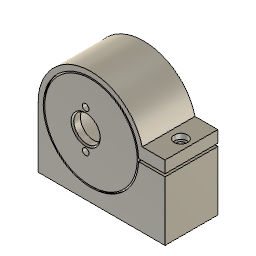
ワインダー量産試作機外装作成前配置 (Autodesk Fusion 360 archive; units mm, degrees)
design "モーターマウント"
Autodesk Fusion 360 part; units mm, degrees
note: some values were not read from the file. Chosen so that the rebuilt part matches the saved one: that a step has no effect. Set by a fixed rule: which sketch regions a step uses.
sketch "スケッチ1" plane through (0, 0, 0) normal (0, 1, 0) x (1, 0, 0)
  line L0 (0, 20) -> (0, 18)
  line L1 (20, -5) -> (28, -5)
  line L2 (20, -5) -> (19.3649, -5)
  line L3 (-20, 23) -> (0, 23)
  line L4 (0, 20) -> (0, 18)
  line L5 (28, 18) -> (28, 23)
  line L6 (28, 23) -> (0, 23)
  line L7 (0, 20) -> (0, 18)
  line L8 (-20, 0) -> (-20, 18)
  arc A0 (-20, 0) -> (19.3649, -5) centre (0, 0) ccw
  line L9 (-20, 18) -> (-20, 23)
  line L10 (28, -0.5) -> (17.9931, -0.5)
  line L11 (17.9931, 0.5) -> (28, 0.5)
  arc A1 (17.9931, 0.5) -> (17.9931, -0.5) centre (0, 0) ccw
  line L12 (28, -5) -> (28, -0.5)
  line L13 (28, 0.5) -> (28, 20)
  dimension "d1" = 36
  dimension "d4" = 5
  constraint coincident A0.centre A1.centre
  constraint vertical L0
  constraint perpendicular L1 L12
  constraint horizontal L3
  constraint vertical L4
  constraint coincident L0.end A1
  constraint vertical L5
  constraint horizontal L6
  constraint vertical L7
  constraint perpendicular L3 L9
  constraint coincident L11.end L12
  constraint perpendicular L11 L12
  constraint collinear L12 L13
  measures "d1" diameter of A1
  measures "d4" distance of L0.end L3.end
extrude "押し出し1" add sketch "スケッチ1" along normal blind 20 makes body 1
sketch "スケッチ2" plane through (0, 0, 5) normal (0, 0, 1) x (-1, 0, 0)
  line L0 (-19.3649, 0) -> (-28, 0)
  line L1 (-28, 0) -> (-28, -20)
  line L2 (-28, -20) -> (-19.3649, -20)
  line L3 (-19.3649, -20) -> (-19.3649, 0)
  circle A0 centre (-24, -10) radius 2.5
  dimension "d7" = 5
  measures "d7" diameter of A0
extrude "押し出し2" cut sketch "スケッチ2" against normal blind 2 contours A0 bodies 1
sketch "スケッチ3" plane through (0, 0, 3) normal (0, 0, 1) x (-1, 0, 0)
  circle A0 centre (-24, -10) radius 2.5
  circle A1 centre (-24, -10) radius 1.5
  dimension "d10" = 3
  constraint concentric A0 A1
  measures "d10" diameter of A1
extrude "押し出し3" cut sketch "スケッチ3" against normal blind 26 contours A1 bodies 1
sketch "スケッチ5" plane through (0, 0, 0) normal (0, 1, 0) x (1, 0, 0)
  line L0 (28, 23) -> (-20, 23)
  line L1 (-20, 23) -> (-20, 19)
  line L2 (-20, 19) -> (28, 19)
  line L3 (28, 19) -> (28, 23)
  constraint horizontal L0
  constraint vertical L1
  constraint horizontal L2
  constraint vertical L3
sketch "スケッチ8" plane through (0, 0, -23) normal (0, 0, -1) x (1, 0, 0)
  line L0 (0, -20) -> (0, 0)
  line L1 (-20, 0) -> (-20, -20)
  line L2 (28, -10) -> (24, -10)
  line L3 (26.8, -8.3834) -> (24, -6.7668)
  line L4 (24, -6.7668) -> (21.2, -8.3834)
  line L5 (21.2, -8.3834) -> (21.2, -11.6166)
  line L6 (21.2, -11.6166) -> (24, -13.2332)
  line L7 (24, -13.2332) -> (26.8, -11.6166)
  line L8 (26.8, -11.6166) -> (26.8, -8.3834)
  line L9 (0, 0) -> (-20, 0)
  line L10 (-20, -20) -> (0, -20)
  point P0 (24, -10)
  dimension "d20" = 4
  dimension "d21" = 2.8
  constraint coincident P0 L2.end
  measures "d20" distance of L2.start P0
  measures "d21" distance of P0 L8
extrude "押し出し6" cut sketch "スケッチ8" against normal blind 15 contours L3 L4 L5 L6 L7 L8 bodies 1
extrude "押し出し7" [no effect]
sketch "スケッチ15" plane through (0, 0, -23) normal (0, 0, -1) x (1, 0, 0)
  line L0 (24, -6.7668) -> (26.8, -8.3834)
  line L1 (26.8, -8.3834) -> (26.8, -11.6166)
  line L2 (26.8, -11.6166) -> (24, -13.2332)
  line L3 (24, -13.2332) -> (21.2, -11.6166)
  line L4 (21.2, -11.6166) -> (21.2, -8.3834)
  line L5 (21.2, -8.3834) -> (24, -6.7668)
  line L6 (28, 0) -> (0, 0)
  line L7 (0, 0) -> (0, -20)
  line L8 (0, -20) -> (28, -20)
  line L9 (28, -20) -> (28, 0)
  point P0 (25, -17)
  point P1 (-17, -17)
  point P2 (-17, -3)
  point P3 (25, -3)
hole "穴2" at (25, 17, -23) at (25, 3, -23) at (-17, 3, -23) at (-17, 17, -23) direction (0, 0, 1) diameter 2.5 depth 5 tip angle 180 bodies 1
sketch "スケッチ1 (2)" plane through (0, 0, 0) normal (0, 1, 0) x (1, 0, 0) in component "モーターマウント(内部) v1"
  circle A0 centre (0, 0) radius 18
  circle A1 centre (-2, 0) radius 13.85
  dimension "d5_1" = 27.7
  constraint coincident A0.centre origin
  measures "d5_1" diameter of A1
extrude "押し出し2'" add sketch "スケッチ1 (2)" along normal blind 20 separate body makes body 2 in component "モーターマウント(内部) v1"
sketch "スケッチ2 (2)" plane through (0, 0, 0) normal (0, 1, 0) x (1, 0, 0) in component "モーターマウント(内部) v1"
  circle A0 centre (-2, 0) radius 13.85
  circle A1 centre (-2, 0) radius 5
  dimension "d8_1" = 27.7
  dimension "d11_1" = 10
  constraint concentric A0 A1
  measures "d8_1" diameter of A0
  measures "d11_1" diameter of A1
extrude "押し出し4" add sketch "スケッチ2 (2)" along normal blind 3 bodies 2 in component "モーターマウント(内部) v1"
sketch "スケッチ3 (2)" plane through (0, 0, 0) normal (0, -1, 0) x (1, 0, 0) in component "モーターマウント(内部) v1"
  circle A0 centre (-2, 0) radius 5
  circle A1 centre (0, 0) radius 18
  circle A2 centre (-2, -7.25) radius 1.25
  line L0 (-2, 0) -> (-2, 7.25)
  circle A3 centre (-2, 7.25) radius 1.25
  point P0 (-2, 0)
  dimension "d14" = 7.25
  dimension "d15" = 2.5
  dimension "d16" = 7.25
  dimension "d17" = 2.5
  constraint coincident P0 A0.centre
  constraint vertical L0
  constraint coincident L0.end A3.centre
  measures "d14" distance of P0 A2.centre
  measures "d15" diameter of A2
  measures "d16" distance of P0 L0.end
  measures "d17" diameter of A3
extrude "押し出し5" cut sketch "スケッチ3 (2)" against normal blind 3 contours A2 | A3 bodies 2 in component "モーターマウント(内部) v1"
chamfer "面取り1" distance 0.5 angle 45 2 edges at (-16.7819, 0, 6.5091) (-6.6616, 0, -1.8081) on bodies 2 in component "モーターマウント(内部) v1"
chamfer "面取り2" distance 0.5 angle 45 2 edges at (-16.7819, 20, 6.5091) (-14.9127, 20, -5.0084) on bodies 2 in component "モーターマウント(内部) v1"
sketch "スケッチ4" plane through (0, 0, 0) normal (0, 1, 0) x (1, 0, 0) in component "モーターマウント(内部) v1"
component "モーターマウント(内部) v1" placed x (1, 0, 0) y (0, 1, 0) z (0, 0, 1) at (0, 0, 0)
